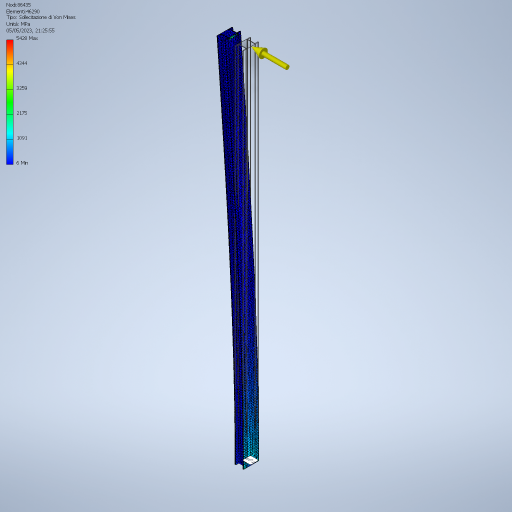
# Autodesk Inventor part: calcolo fem
Saved by Autodesk Inventor 2023 (Build 270158000, 158)
## iProperties
Created: 2023-05-05
Part Number: calcolo fem
Material: Generico
Document SubType Name: Modeling
Designer: Admin
Density: 1 g/cm^3
Appearance: Default
Author: Admin
Autodesk Inventor part; units mm, degrees
ref_plane "YZ Plane" through (0, 0, 0) normal (1, 0, 0) x (0, 1, 0)
ref_plane "XZ Plane" through (0, 0, 0) normal (0, 1, 0) x (-1, 0, 0)
ref_plane "XY Plane" through (0, 0, 0) normal (0, 0, 1) x (1, 0, 0)
sketch "Schizzo1" plane through (0, 0, 0) normal (0, 1, 0) x (-1, 0, 0)
  line L0 (14.898, -21.6987) -> (14.898, -31.6987)
  line L1 (-8.102, -21.6987) -> (-8.102, -31.6987)
  line L2 (-8.102, -31.6987) -> (-11.102, -31.6987)
  line L3 (-8.102, -21.6987) -> (14.898, -21.6987)
  line L4 (-10.3886, -19.6987) -> (17.0348, -19.6987)
  line L5 (14.898, -31.6987) -> (17.898, -31.6987)
  line L6 (17.898, -6.6987) -> (-17.7474, -6.6987) construction
  line L7 (-10.3886, 6.3013) -> (-10.3886, -19.6987)
  line L8 (17.0348, 6.3013) -> (-10.3886, 6.3013)
  line L9 (-10.3886, -19.6987) -> (17.0348, 6.3013) construction
  line L10 (17.0348, -19.6987) -> (-10.3886, 6.3013) construction
  line L11 (14.898, 8.3013) -> (-8.102, 8.3013)
  line L12 (-11.102, -31.6987) -> (-11.102, 18.3013)
  line L13 (17.898, -31.6987) -> (17.898, 18.3013)
  line L14 (-11.102, 18.3013) -> (-8.102, 18.3013)
  line L15 (14.898, 18.3013) -> (14.898, 8.3013)
  line L16 (17.898, 18.3013) -> (14.898, 18.3013)
  line L17 (17.0348, -19.6987) -> (17.0348, 6.3013)
  line L18 (-8.102, 18.3013) -> (-8.102, 8.3013)
  line L19 (17.2869, 17.8522) -> (15.509, 17.8522)
  line L20 (15.509, 17.8522) -> (15.509, 8.7505)
  line L21 (15.509, 8.7505) -> (17.2869, 8.7505)
  line L22 (17.2869, 8.7505) -> (17.2869, 17.8522)
  line L23 (17.2869, 17.8522) -> (15.509, 8.7505) construction
  line L24 (15.509, 17.8522) -> (17.2869, 8.7505) construction
  line L25 (17.2869, -22.1954) -> (15.509, -22.1954)
  line L26 (15.509, -22.1954) -> (15.509, -31.202)
  line L27 (15.509, -31.202) -> (17.2869, -31.202)
  line L28 (17.2869, -31.202) -> (17.2869, -22.1954)
  line L29 (17.2869, -22.1954) -> (15.509, -31.202) construction
  line L30 (15.509, -22.1954) -> (17.2869, -31.202) construction
  line L31 (-8.5206, -22.1954) -> (-10.6835, -22.1954)
  line L32 (-10.6835, -22.1954) -> (-10.6835, -31.202)
  line L33 (-10.6835, -31.202) -> (-8.5206, -31.202)
  line L34 (-8.5206, -31.202) -> (-8.5206, -22.1954)
  line L35 (-8.5206, -22.1954) -> (-10.6835, -31.202) construction
  line L36 (-10.6835, -22.1954) -> (-8.5206, -31.202) construction
  line L37 (-8.5206, 17.8522) -> (-10.6835, 17.8522)
  line L38 (-10.6835, 17.8522) -> (-10.6835, 8.7505)
  line L39 (-10.6835, 8.7505) -> (-8.5206, 8.7505)
  line L40 (-8.5206, 8.7505) -> (-8.5206, 17.8522)
  line L41 (-8.5206, 17.8522) -> (-10.6835, 8.7505) construction
  line L42 (-10.6835, 17.8522) -> (-8.5206, 8.7505) construction
  line L43 (-10.2389, 6.9058) -> (17.0348, 6.9058)
  line L44 (17.0348, 6.9058) -> (17.0348, 7.7637)
  line L45 (17.0348, 7.7637) -> (-10.2389, 7.7637)
  line L46 (-10.2389, 7.7637) -> (-10.2389, 6.9058)
  line L47 (-10.2389, 6.9058) -> (17.0348, 7.7637) construction
  line L48 (17.0348, 6.9058) -> (-10.2389, 7.7637) construction
  line L49 (-10.2389, -21.0418) -> (17.0348, -21.0418)
  line L50 (17.0348, -21.0418) -> (17.0348, -20.3019)
  line L51 (17.0348, -20.3019) -> (-10.2389, -20.3019)
  line L52 (-10.2389, -20.3019) -> (-10.2389, -21.0418)
  line L53 (-10.2389, -21.0418) -> (17.0348, -20.3019) construction
  line L54 (17.0348, -21.0418) -> (-10.2389, -20.3019) construction
  point P0 (0, 0)
  point P1 (0, 0)
  point P2 (3.3231, -6.6987)
  point P3 (16.398, 13.3013)
  point P4 (16.398, -26.6987)
  point P5 (-9.602, -26.6987)
  point P6 (-9.602, 13.3013)
  point P7 (3.398, 7.3347)
  point P8 (3.398, -20.6718)
  dimension "d0" = 50
  dimension "d1" = 23
  dimension "d2" = 3
  dimension "d3" = 10
  dimension "d4" = 10
  dimension "d5" = 10
  dimension "d6" = 2
  dimension "d7" = 2
  constraints: 110 end point, 20 parallel, 15 midpoint, 14 perpendicular, 10 horizontal, 6 point on line, 1 collinear
  measures "d0" distance of L13.start L13.end
  measures "d1" distance of L1.start L0.start
  measures "d2" distance of L0.end L13.start
  measures "d3" distance of L18.start L11.end
  measures "d4" distance of L1.start L1.end
  measures "d5" distance of L0.start L0.end
  measures "d6" distance between parallel lines of L8 L11
  measures "d7" distance between parallel lines of L3 L4
extrude "Estrusione1" add sketch "Schizzo1" along normal blind 1200
